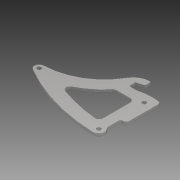
# Autodesk Inventor part: Накладка_4.1.4_3.1
Saved by Autodesk Inventor 2016 (Build 200138000, 138)
## iProperties
Created: 2020-03-12
Part Number: Накладка_4.1.4_3.1
Material: Поликарбонат, прозрачный
Document SubType Name: Modeling
Designer: Рябов
Density: 1.2 g/cm^3
Appearance: Поликарбонат — прозрачный
Mass: 4.25787 g
Surface Area: 43.0708 cm^2
Volume: 3.54822 cm^3
Author: Рябов
Autodesk Inventor part; units mm, degrees
ref_plane "YZ Plane" through (0, 0, 0) normal (1, 0, 0) x (0, 1, 0)
ref_plane "XZ Plane" through (0, 0, 0) normal (0, 1, 0) x (-1, 0, 0)
ref_plane "XY Plane" through (0, 0, 0) normal (0, 0, 1) x (1, 0, 0)
sketch "Эскиз1" plane through (0, 0, 0) normal (0, 0, 1) x (1, 0, 0)
  circle A0 centre (6.4823, -1.4624) radius 1.65
  circle A1 centre (6.4823, -40.9716) radius 1.65 construction
  arc A2 (-57.7734, 9.189) -> (-62.7021, 3.6942) centre (-59.7433, 5.998) ccw construction
  circle A3 centre (-59.7433, 5.998) radius 1.65 construction
  line L0 (-4.1893, 7.0157) -> (-4.1893, 7.0357) construction
  line L1 (-4.1893, 7.0357) -> (-3.1893, 7.0357) construction
  line L2 (-3.1893, 7.0357) -> (-3.1893, 7.0157) construction
  line L3 (-3.1893, 7.0157) -> (-1.1893, 7.0157) construction
  line L4 (-1.1893, 7.0157) -> (-1.1893, 7.0357) construction
  line L5 (-1.1893, 7.0357) -> (0.8107, 7.0357) construction
  line L6 (0.8107, 7.0357) -> (0.8107, 6.6351) construction
  line L7 (0.8107, 6.6351) -> (-1.1893, 6.6351) construction
  line L8 (-1.1893, 6.6351) -> (-1.1893, 6.6551) construction
  line L9 (-1.1893, 6.6551) -> (-3.1893, 6.6551) construction
  line L10 (-3.1893, 6.6551) -> (-3.1893, 6.6351) construction
  line L11 (-3.1893, 6.6351) -> (-4.1893, 6.6351) construction
  line L12 (-4.1893, 6.6351) -> (-4.1893, 6.6551) construction
  line L13 (-4.1893, 6.6551) -> (-6.1893, 6.6551) construction
  line L14 (-6.1893, 6.6551) -> (-6.1893, 6.6351) construction
  line L15 (-6.1893, 6.6351) -> (-7.1893, 6.6351) construction
  line L16 (-7.1893, 6.6351) -> (-7.1893, 6.6551) construction
  line L17 (-7.1893, 6.6551) -> (-9.1893, 6.6551) construction
  line L18 (-9.1893, 6.6551) -> (-9.1893, 6.6351) construction
  line L19 (-9.1893, 6.6351) -> (-11.1893, 6.6351) construction
  line L20 (-11.1893, 6.6351) -> (-11.1893, 7.0357) construction
  line L21 (-11.1893, 7.0357) -> (-9.1893, 7.0357) construction
  line L22 (-9.1893, 7.0357) -> (-9.1893, 7.0157) construction
  line L23 (-9.1893, 7.0157) -> (-7.1893, 7.0157) construction
  line L24 (-7.1893, 7.0157) -> (-7.1893, 7.0357) construction
  line L25 (-7.1893, 7.0357) -> (-6.1893, 7.0357) construction
  line L26 (-6.1893, 7.0357) -> (-6.1893, 7.0157) construction
  line L27 (-6.1893, 7.0157) -> (-4.1893, 7.0157) construction
  line L28 (-7.6643, 167.4795) -> (-7.6643, 168.8316) construction
  line L29 (-7.6643, 168.8316) -> (-7.1353, 168.8316) construction
  spline S0 degree 3 poles (-7.1353, 168.8316) (-7.0277, 168.8151) (-6.9171, 168.7981) (-6.7021, 168.7651) (-6.5903, 168.748) (-6.4827, 168.7315) knots 0 0 0 0 0.501572 0.501572 1 1 1 1 construction
  line L30 (-6.4827, 168.7315) -> (-3.8958, 168.7315) construction
  spline S1 degree 3 poles (-3.8958, 168.7315) (-3.7882, 168.748) (-3.6765, 168.7651) (-3.4615, 168.7981) (-3.3509, 168.8151) (-3.2433, 168.8316) knots 0 0 0 0 0.498467 0.498467 1 1 1 1 construction
  line L31 (-3.2433, 168.8316) -> (-2.7143, 168.8316) construction
  line L32 (-2.7143, 168.8316) -> (-2.7143, 167.4795) construction
  line L33 (-2.7143, 167.4795) -> (-3.7643, 167.4795) construction
  line L34 (-3.7643, 167.4795) -> (-3.7643, 167.3293) construction
  line L35 (-3.7643, 167.3293) -> (-4.6551, 167.3293) construction
  spline S2 degree 3 poles (-4.6551, 167.3293) (-4.6545, 167.3543) (-4.654, 167.3794) (-4.6529, 167.4294) (-4.6524, 167.4545) (-4.6519, 167.4795) knots 0 0 0 0 0.500007 0.500007 1 1 1 1 construction
  line L36 (-4.6519, 167.4795) -> (-5.7266, 167.4795) construction
  spline S3 degree 3 poles (-5.7266, 167.4795) (-5.7261, 167.4545) (-5.7256, 167.4294) (-5.7245, 167.3794) (-5.724, 167.3543) (-5.7235, 167.3293) knots 0 0 0 0 0.5 0.5 1 1 1 1 construction
  line L37 (-5.7235, 167.3293) -> (-6.6143, 167.3293) construction
  line L38 (-6.6143, 167.3293) -> (-6.6143, 167.4795) construction
  line L39 (-6.6143, 167.4795) -> (-7.6643, 167.4795) construction
  line L40 (0.8107, 166.7784) -> (-11.1893, 166.7784) construction
  line L41 (-11.1893, 166.7784) -> (-11.1893, 167.179) construction
  line L42 (-11.1893, 167.179) -> (-4.3383, 167.179) construction
  spline S4 degree 3 poles (-4.3383, 167.179) (-4.3383, 167.1792) (-4.3383, 167.1794) (-4.3383, 167.1797) (-4.3383, 167.1799) (-4.3383, 167.18) knots 0 0 0 0 0.499986 0.499986 1 1 1 1 construction
  line L43 (-4.3383, 167.18) -> (-4.2964, 167.18) construction
  spline S5 degree 3 poles (-4.2964, 167.18) (-4.2964, 167.1799) (-4.2964, 167.1797) (-4.2963, 167.1794) (-4.2963, 167.1792) (-4.2963, 167.179) knots 0 0 0 0 0.500002 0.500002 1 1 1 1 construction
  line L44 (-4.2963, 167.179) -> (0.8107, 167.179) construction
  line L45 (0.8107, 167.179) -> (0.8107, 166.7784) construction
  line L46 (-11.1893, 6.6251) -> (0.8107, 6.6251) construction
  spline S6 degree 3 poles (0.8107, 6.6251) (0.8107, 6.4396) (0.7674, 6.2212) (0.6255, 5.8786) (0.5021, 5.6936) (0.2685, 5.4598) (0.1339, 5.3598) (-0.0029, 5.2893) knots 0 0 0 0 0.359545 0.359545 0.718791 0.718791 1 1 1 1 construction
  spline S7 degree 3 poles (-0.0029, 5.2893) (-0.2886, 5.142) (-0.5748, 5.01) (-1.5002, 4.6264) (-2.2318, 4.3978) (-3.7268, 4.1001) (-4.4903, 4.0311) (-5.1893, 4.0311) (-5.8883, 4.0311) (-6.6517, 4.1001) (-8.1467, 4.3978) (-8.8784, 4.6264) (-9.8038, 5.01) (-10.0899, 5.142) (-10.3757, 5.2893) knots -0.510232 -0.510232 -0.510232 -0.510232 -0.41941 -0.41941 -0.209705 -0.209705 0 0 0 0.209705 0.209705 0.41941 0.41941 0.510232 0.510232 0.510232 0.510232 construction
  spline S8 degree 3 poles (-10.3757, 5.2893) (-10.5125, 5.3598) (-10.6471, 5.4598) (-10.8806, 5.6936) (-11.0041, 5.8786) (-11.1459, 6.2212) (-11.1893, 6.4396) (-11.1893, 6.6251) knots 0 0 0 0 0.281209 0.281209 0.640455 0.640455 1 1 1 1 construction
  line L47 (0.8107, 167.1891) -> (-11.1893, 167.1891) construction
  spline S9 degree 3 poles (-11.1893, 167.1891) (-11.1893, 167.3746) (-11.1459, 167.5929) (-11.0041, 167.9356) (-10.8806, 168.1206) (-10.6471, 168.3544) (-10.5125, 168.4544) (-10.3757, 168.5249) knots 0 0 0 0 0.359545 0.359545 0.718791 0.718791 1 1 1 1 construction
  spline S10 degree 3 poles (-10.3757, 168.5249) (-10.0899, 168.6722) (-9.8038, 168.8041) (-8.8784, 169.1877) (-8.1467, 169.4164) (-6.6517, 169.714) (-5.8883, 169.7831) (-5.1893, 169.7831) (-4.4903, 169.7831) (-3.7268, 169.714) (-2.2318, 169.4164) (-1.5002, 169.1877) (-0.5748, 168.8041) (-0.2886, 168.6722) (-0.0029, 168.5249) knots -0.510232 -0.510232 -0.510232 -0.510232 -0.41941 -0.41941 -0.209705 -0.209705 0 0 0 0.209705 0.209705 0.41941 0.41941 0.510232 0.510232 0.510232 0.510232 construction
  spline S11 degree 3 poles (-0.0029, 168.5249) (0.1339, 168.4544) (0.2685, 168.3544) (0.5021, 168.1206) (0.6255, 167.9356) (0.7674, 167.5929) (0.8107, 167.3746) (0.8107, 167.1891) knots 0 0 0 0 0.281209 0.281209 0.640455 0.640455 1 1 1 1 construction
  line L48 (0.8107, 7.0357) -> (-11.1893, 7.0357) construction
  line L49 (-11.1893, 7.0357) -> (-11.1893, 9.0391) construction
  line L50 (-11.1893, 9.0391) -> (0.8107, 9.0391) construction
  line L51 (0.8107, 9.0391) -> (0.8107, 7.0357) construction
  line L52 (-11.1893, 166.7784) -> (0.8107, 166.7784) construction
  line L53 (0.8107, 166.7784) -> (0.8107, 164.7751) construction
  line L54 (0.8107, 164.7751) -> (-11.1893, 164.7751) construction
  line L55 (-11.1893, 164.7751) -> (-11.1893, 166.7784) construction
  line L56 (8.8107, -34.9344) -> (8.8107, -18.7776) construction
  arc A4 (10.3107, -17.2776) -> (8.8107, -18.7776) centre (10.3107, -18.7776) ccw construction
  line L57 (10.3107, -17.2776) -> (10.8107, -17.2776) construction
  arc A5 (10.8107, -17.2776) -> (13.3107, -14.7776) centre (10.8107, -14.7776) ccw construction
  arc A6 (8.8107, -34.9344) -> (10.3107, -36.4344) centre (10.3107, -34.9344) ccw construction
  line L58 (10.8107, -36.4344) -> (10.3107, -36.4344) construction
  arc A7 (13.3107, -38.9344) -> (10.8107, -36.4344) centre (10.8107, -38.9344) ccw construction
  circle A8 centre (6.4823, -37.9624) radius 43.5897 construction
  circle A9 centre (6.4823, -37.9624) radius 50.2137 construction
  line L59 (-5.1893, 7.0357) -> (-5.1893, 4.0357) construction
  line L60 (-5.1893, 11.659) -> (-5.1893, 14.7497)
  arc A10 (-5.9418, 10.6901) -> (-10.3994, 9.3285) centre (6.4823, -37.9624) ccw
  circle A11 centre (-59.7433, -19.7124) radius 1.65
  line L61 (-72.3399, -9.8595) -> (-95.7506, 3.6566) construction
  line L62 (-59.7433, -19.7124) -> (-59.7433, -1.4624) construction
  line L63 (-11.1893, 9.0391) -> (-11.1893, 7.6248) construction
  line L64 (-10.1893, 4.0357) -> (-5.3249, 4.0357)
  arc A12 (11.0741, 5.3849) -> (-5.0601, 4.0714) centre (6.4823, -37.9624) ccw
  line L65 (13.3107, 2.8988) -> (13.3107, -14.7776)
  line L66 (0.8107, -46.4344) -> (13.3107, -46.4344) construction
  arc A13 (-61.642, -22.9461) -> (10.9586, -42.6846) centre (10.9586, 100.7017) ccw
  line L67 (-61.642, -22.9461) -> (-59.7504, -24.0568) construction
  circle A14 centre (6.4823, -37.9624) radius 52.481 construction
  arc A15 (-10.3994, 9.3285) -> (-11.1893, 7.6248) centre (-10.4822, 8.3319) ccw
  line L68 (-11.1893, 9.0391) -> (-10.4822, 8.3319) construction
  arc A16 (-11.1893, 5.0357) -> (-10.1893, 4.0357) centre (-10.1893, 5.0357) ccw
  arc A17 (-5.3249, 4.0357) -> (-5.0601, 4.0714) centre (-5.3249, 5.0357) ccw
  arc A18 (13.3107, 2.8988) -> (11.0741, 5.3849) centre (10.8107, 2.8988) ccw
  arc A19 (-5.1893, 14.7497) -> (-6.1893, 15.7497) centre (-6.1893, 14.7497) ccw
  arc A20 (-5.9418, 10.6901) -> (-5.1893, 11.659) centre (-6.1893, 11.659) ccw
  line L69 (0.8107, -29.02) -> (0.8107, -6.9643)
  line L70 (-13.1559, -3.9643) -> (-2.1893, -3.9643)
  line L71 (0.8107, 32.412) -> (0.8107, -57.5372) construction
  arc A21 (-33.9311, -19.5241) -> (-15.4341, -5.0125) centre (-60.9999, 34.023) ccw
  arc A22 (-33.5794, -25.0292) -> (-2.4918, -32.0047) centre (10.9586, 100.7017) ccw
  arc A23 (0.8107, -6.9643) -> (-2.1893, -3.9643) centre (-2.1893, -6.9643) ccw
  arc A24 (-13.1559, -3.9643) -> (-15.4341, -5.0125) centre (-13.1559, -6.9643) ccw
  arc A25 (-33.9311, -19.5241) -> (-33.5794, -25.0292) centre (-32.5777, -22.2014) ccw
  arc A26 (-2.4918, -32.0047) -> (0.8107, -29.02) centre (-2.1893, -29.02) ccw
  line L72 (10.8107, -37.8324) -> (10.3107, -37.8324)
  line L73 (8.8107, -36.3324) -> (8.8107, -24.3324)
  line L74 (10.3107, -22.8324) -> (10.8107, -22.8324)
  line L75 (13.3107, -20.3324) -> (13.3107, -14.7776)
  arc A27 (10.8107, -22.8324) -> (13.3107, -20.3324) centre (10.8107, -20.3324) ccw
  arc A28 (13.3107, -40.3324) -> (10.8107, -37.8324) centre (10.8107, -40.3324) ccw
  arc A29 (10.3107, -22.8324) -> (8.8107, -24.3324) centre (10.3107, -24.3324) ccw
  arc A30 (8.8107, -36.3324) -> (10.3107, -37.8324) centre (10.3107, -36.3324) ccw
  circle A31 centre (6.4823, -37.9624) radius 1.65
  arc A32 (10.9586, -42.6846) -> (13.3107, -40.3324) centre (10.9586, -40.3324) ccw
  line L76 (19.1681, -42.6846) -> (-36.8509, -42.6846) construction
  arc A33 (-10.3994, 9.3285) -> (-11.1893, 9.0391) centre (6.4823, -37.9624) ccw construction
  line L77 (-11.1893, 7.6248) -> (-11.1893, 5.0357)
  arc A34 (-59.8309, -15.9634) -> (-17.6428, 9.1199) centre (-60.9999, 34.023) ccw
  arc A35 (-59.8309, -15.9634) -> (-61.642, -22.9461) centre (-59.7433, -19.7124) ccw
  arc A36 (-5.1667, 16.0085) -> (-12.0803, 14.0375) centre (6.4823, -37.9624) ccw construction
  arc A37 (-6.1893, 15.7497) -> (-17.6428, 9.1199) centre (-6.1893, 2.5413) ccw
  line L78 (-6.1893, 15.7497) -> (-16.5229, 15.7497) construction
  line L79 (6.4823, -1.4624) -> (6.4823, -37.9624) construction
  line L80 (15.3107, -35.3592) -> (15.3107, -25.3056)
  point P0 (0, 0)
  point P1 (-5.1893, 10.8761)
  point P2 (-5.1893, 16.0036)
  point P3 (-5.1893, 9.0391)
  point P4 (13.3107, 5.0892)
  point P5 (13.3107, -46.4344)
  point P6 (0.8107, -42.325)
  point P7 (-35.4501, -6.404)
  point P8 (-57.8683, -18.2148)
  point P9 (-5.1893, 13.2043)
  point P10 (-8.669, 12.284)
  point P11 (0.8107, -32.298)
  point P12 (0.8107, -3.9643)
  point P13 (-14.5567, -3.9643)
  point P14 (0.8107, -32.298)
  point P15 (8.8107, -37.8324)
  point P16 (8.8107, -22.8324)
  point P17 (13.3107, -22.8324)
  point P18 (6.4823, -19.7124)
  point P19 (15.3107, -30.3324)
  point P20 (8.8107, -30.3324)
  dimension "d0" = 3
  dimension "d10" = 60
  dimension "d12" = 45
  dimension "d13" = 2
  dimension "d14" = 1
  dimension "d17" = 1
  dimension "d23" = 10
  dimension "d25" = 8
  dimension "d26" = 3
  dimension "d27" = 15
  dimension "d33" = 36.5
  dimension "d36" = 3
  dimension "d39" = 7.5
  dimension "d41" = 10
  dimension "d42" = 5
  dimension "d46" = 50
  dimension "d48" = 5
  constraints: 151 end point, 66 point on circle, 38 tangent, 34 horizontal, 31 vertical, 30 centre point, 23 point on line, 12 equal radius, 6 midpoint, 5 perpendicular, 4 coincident, 4 vertical alignment, 3 concentric, 2 horizontal alignment, 1 collinear, 98 other
  measures "d0" distance of L59.start L59.end
  measures "d10" angle of L62 L61
  measures "d12" angle of L63 L68
  measures "d13" diameter of A15
  measures "d14" radius of A16
  measures "d17" radius of A19
  measures "d23" radial gap between concentric circles of A13 A22
  measures "d25" distance between parallel lines of L70 L64
  measures "d26" radius of A23
  measures "d27" distance between parallel lines of L72 L74
  measures "d33" distance of A8.centre L79.start
  measures "d39" diameter of A35
  measures "d41" radial gap between concentric circles of A34 A21
  measures "d42" radial gap between concentric circles of A10 A36
  measures "d46" radius of A34
extrude "Выдавливание1" add sketch "Эскиз1" against normal blind 2
fillet "Сопряжение1" radius 1 2 edges at (-11.1893, 7.6248, -1) (-10.3994, 9.3285, -1)
delete faces "Удаление грани1" heal yes whole lump no faces at (13.1379, -39.4191, -1.3333) (10.6441, -37.8324, -0.6667) (9.7627, -37.7287, -1.3333) (12.2836, -42.2759, -1.3333)
sketch "Эскиз2" plane through (-10.1893, 4.0357, 0) normal (0, 0, 1) x (1, 0, 0)
  line L0 (19, -46.7042) -> (19, -28.3682) projected
  arc A0 (20.5, -26.8682) -> (19, -28.3682) centre (20.5, -28.3682) ccw projected
  line L1 (20.5, -26.8682) -> (21, -26.8682) projected
  arc A1 (21, -26.8682) -> (23.5, -24.3682) centre (21, -24.3682) ccw projected
  line L2 (23.5, -24.3682) -> (23.5, -1.137) projected
  arc A2 (23.5, -1.137) -> (21.2634, 1.3491) centre (21, -1.137) ccw projected
  arc A3 (21.2634, 1.3491) -> (5.1292, 0.0357) centre (16.6716, -41.9981) ccw projected
  arc A4 (4.8644, 0) -> (5.1292, 0.0357) centre (4.8644, 1) ccw projected
  line L3 (4.8644, 0) -> (0, 0) projected
  arc A5 (-1, 1) -> (0, 0) centre (0, 1) ccw projected
  line L4 (-1, 1) -> (-1, 3.2542) projected
  arc A6 (-1, 3.2542) -> (-1.1464, 3.7752) centre (-2, 3.2542) ccw projected
  arc A7 (-0.3353, 5.2953) -> (-1.1464, 3.7752) centre (-0.2929, 4.2962) ccw projected
  arc A8 (-0.3353, 5.2953) -> (-0.0448, 5.3514) centre (-0.3777, 6.2944) ccw projected
  arc A9 (4.2474, 6.6543) -> (-0.0448, 5.3514) centre (16.6716, -41.9981) ccw projected
  arc A10 (4.2474, 6.6543) -> (5, 7.6232) centre (4, 7.6232) ccw projected
  line L5 (5, 7.6232) -> (5, 10.7139) projected
  arc A11 (5, 10.7139) -> (4, 11.7139) centre (4, 10.7139) ccw projected
  arc A12 (4, 11.7139) -> (-7.4535, 5.0841) centre (4, -1.4944) ccw projected
  arc A13 (-49.6417, -19.9991) -> (-7.4535, 5.0841) centre (-50.8106, 29.9872) ccw projected
  arc A14 (-49.6417, -19.9991) -> (-51.4527, -26.9819) centre (-49.554, -23.7481) ccw projected
  arc A15 (-51.4527, -26.9819) -> (19, -46.7042) centre (21.1478, 96.666) ccw projected
  arc A16 (-2.9666, -8) -> (-5.2449, -9.0482) centre (-2.9666, -11) ccw projected
  line L6 (-2.9666, -8) -> (8, -8) projected
  arc A17 (11, -11) -> (8, -8) centre (8, -11) ccw projected
  line L7 (11, -11) -> (11, -33.0557) projected
  arc A18 (7.6975, -36.0404) -> (11, -33.0557) centre (8, -33.0557) ccw projected
  arc A19 (-23.3901, -29.065) -> (7.6975, -36.0404) centre (21.1478, 96.666) ccw projected
  arc A20 (-23.7419, -23.5598) -> (-23.3901, -29.065) centre (-22.3884, -26.2372) ccw projected
  arc A21 (-23.7419, -23.5598) -> (-5.2449, -9.0482) centre (-50.8106, 29.9872) ccw projected
  circle A22 centre (16.6716, -41.9981) radius 1.65 projected
  circle A23 centre (-49.554, -23.7481) radius 1.65 projected
  circle A24 centre (16.6716, -5.4981) radius 1.65 projected
  arc A25 (16.5215, -46.6457) -> (19, -46.0231) centre (16.6716, -41.9981) ccw
  arc A26 (-51.4527, -26.9819) -> (19, -46.7042) centre (21.1478, 96.666) ccw projected
  arc A27 (19, -46.0231) -> (19, -37.9731) centre (16.6716, -41.9981) ccw
  point P0 (10.1893, -4.0357)
  constraints: 5 point on circle, 2 centre point, 2 point on line, 1 coincident, 1 tangent
extrude "Выдавливание2" cut sketch "Эскиз2" against normal blind 10 contours A15 A25 L0
extrude "Выдавливание3" add sketch "Эскиз2" against normal up to surface (2 mm away) contours L0 A27
fillet "Сопряжение2" radius 3 1 edges at (8.8107, -33.9373, -1)
